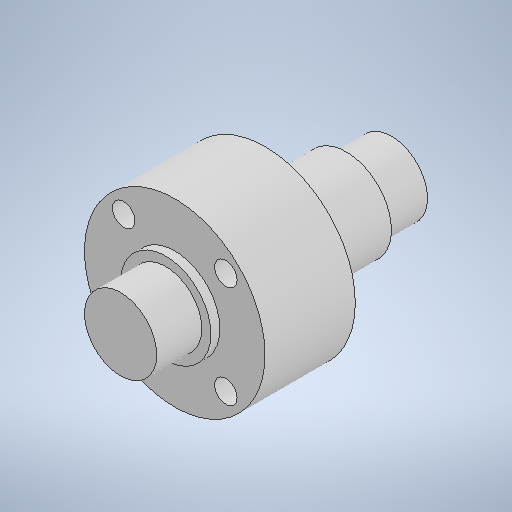
# Autodesk Inventor part: AR20.0_wheel-shaft
Saved by Autodesk Inventor 2025 (Build 290162000, 162)
## iProperties
Created: 2024-07-17
Part Number: AR20.0_wheel-shaft
Material: 一般
Document SubType Name: Modeling
Designer: 8326d
Density: 1 g/cm^3
Appearance: 既定
Author: 8326d
Autodesk Inventor part; units mm, degrees
ref_plane "YZ Plane" through (0, 0, 0) normal (1, 0, 0) x (0, 1, 0)
ref_plane "XZ Plane" through (0, 0, 0) normal (0, 1, 0) x (-1, 0, 0)
ref_plane "XY Plane" through (0, 0, 0) normal (0, 0, 1) x (1, 0, 0)
sketch "スケッチ1" plane through (0, 0, 0) normal (0, 0, 1) x (1, 0, 0)
  circle A0 centre (0, 0) radius 10
  dimension "d0" = 20
  constraints: 1 centre point, 1 coincident
  measures "d0" diameter of A0
extrude "押し出し1" add sketch "スケッチ1" along normal blind 10
sketch "スケッチ2" plane through (0, 0, 10) normal (0, 0, 1) x (1, 0, 0)
  circle A0 centre (0, 0) radius 5
  dimension "d3" = 10
  constraints: 1 centre point, 1 coincident
  measures "d3" diameter of A0
extrude "押し出し2" add sketch "スケッチ2" along normal blind 1
sketch "スケッチ3" plane through (0, 0, 11) normal (0, 0, 1) x (1, 0, 0)
  circle A0 centre (0, 0) radius 4
  dimension "d6" = 8
  constraints: 1 centre point, 1 coincident
  measures "d6" diameter of A0
extrude "押し出し3" add sketch "スケッチ3" along normal blind 5
sketch "スケッチ4" plane through (0, 0, 0) normal (0, 0, -1) x (-1, 0, 0)
  circle A0 centre (0, 0) radius 5
  dimension "d9" = 10
  constraints: 1 centre point, 1 coincident
  measures "d9" diameter of A0
extrude "押し出し4" add sketch "スケッチ4" along normal blind 9
sketch "スケッチ5" plane through (0, 0, -9) normal (0, 0, -1) x (-1, 0, 0)
  circle A0 centre (0, 0) radius 4
  dimension "d12" = 8
  constraints: 1 centre point, 1 coincident
  measures "d12" diameter of A0
extrude "押し出し5" add sketch "スケッチ5" along normal blind 5
sketch "スケッチ6" plane through (0, 0, 0) normal (0, 0, -1) x (-1, 0, 0)
  circle A0 centre (0, 0) radius 8 construction
  line L0 (-5.6569, -5.6569) -> (5.6569, -5.6569) construction
  line L1 (5.6569, -5.6569) -> (5.6569, 5.6569) construction
  line L2 (5.6569, 5.6569) -> (-5.6569, 5.6569) construction
  line L3 (-5.6569, 5.6569) -> (-5.6569, -5.6569) construction
  line L4 (-5.6569, -5.6569) -> (5.6569, 5.6569) construction
  line L5 (5.6569, -5.6569) -> (-5.6569, 5.6569) construction
  dimension "d15" = 16
  constraints: 12 end point, 2 midpoint, 2 parallel, 2 perpendicular, 1 coincident, 1 horizontal, 3 other
hole "穴1" at (-5.6569, 5.6569, 0) at (5.6569, 5.6569, 0) at (5.6569, -5.6569, 0) at (-5.6569, -5.6569, 0) direction (0, 0, 1) diameter 2.5 end through all
